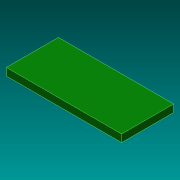
# Autodesk Inventor part: スマホ
Saved by Autodesk Inventor 2015 (Build 190159000, 159)
## iProperties
Created: 2016-05-04
Part Number: スマホ
Material: 一般
Document SubType Name: Modeling
Designer: hiroaki
Mass: 160 g
Surface Area: 327.4 cm^2
Volume: 138.4 cm^3
Density: 1.15607 g/cm^3
Appearance: 濃い緑
Author: hiroaki
Autodesk Inventor part; units mm, degrees
ref_plane "YZ Plane" through (0, 0, 0) normal (1, 0, 0) x (0, 1, 0)
ref_plane "XZ Plane" through (0, 0, 0) normal (0, 1, 0) x (-1, 0, 0)
ref_plane "XY Plane" through (0, 0, 0) normal (0, 0, 1) x (1, 0, 0)
sketch "スケッチ1" plane through (0, 0, 0) normal (0, 0, 1) x (1, 0, 0)
  line L0 (-77.5, -35) -> (77.5, -35)
  line L1 (77.5, -35) -> (77.5, 35)
  line L2 (77.5, 35) -> (-77.5, 35)
  line L3 (-77.5, 35) -> (-77.5, -35)
  line L4 (-77.5, -35) -> (77.5, 35) construction
  line L5 (77.5, -35) -> (-77.5, 35) construction
  point P0 (0, 0)
  dimension "d0" = 155
  dimension "d1" = 70
  constraints: 12 end point, 2 midpoint, 2 parallel, 1 horizontal, 1 perpendicular
  measures "d0" distance of L1.end L2.end
  measures "d1" distance of L0.end L1.end
extrude "押し出し1" add sketch "スケッチ1" along normal blind 5
mirror "ミラー1" about plane through (0, 0, 0) normal (0, 0, -1) of "押し出し1"
